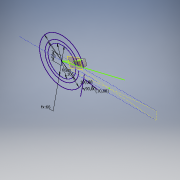
# Autodesk Inventor part: end_stop_plug_v3
Saved by Autodesk Inventor 2016 (Build 200138000, 138)
## iProperties
Created: 2017-11-21
Part Number: end_stop_plug_v3
Material: Generic
Document SubType Name: Modeling
Designer: mbouhier
Density: 1 g/cm^3
Appearance: Default
Author: mbouhier
Autodesk Inventor part; units mm, degrees
ref_plane "YZ Plane" through (0, 0, 0) normal (1, 0, 0) x (0, 1, 0)
ref_plane "XZ Plane" through (0, 0, 0) normal (0, 1, 0) x (-1, 0, 0)
ref_plane "XY Plane" through (0, 0, 0) normal (0, 0, 1) x (1, 0, 0)
sketch "Sketch1" plane through (0, 0, 0) normal (0, 1, 0) x (-1, 0, 0)
  arc A0 (-33, 0) -> (-32.0949, 7.6757) centre (0, 0) ccw
  arc A1 (-40, 0) -> (-38.9029, 9.3039) centre (0, 0) ccw
  arc A2 (-53, 0) -> (-51.5464, 12.3276) centre (0, 0) ccw
  line L0 (-85, 0) -> (100, 0) construction
  line L1 (-226, 10) -> (0, 10) construction
  line L2 (0, 10) -> (0, -10) construction
  line L3 (0, -10) -> (-226, -10) construction
  line L4 (-226, -10) -> (-226, 10) construction
  line L5 (-226, 10) -> (0, -10) construction
  line L6 (0, 10) -> (-226, -10) construction
  line L7 (-52.0481, -10) -> (-44.1646, -51.032)
  line L8 (-38.9029, 9.3039) -> (-32.0949, 7.6757)
  line L9 (-52.0481, -10) -> (-84.6485, -16.2635)
  circle A3 centre (0, 0) radius 33 construction
  line L10 (0, 0) -> (-30.9399, 11.477) construction
  line L11 (-35.5594, 18.3175) -> (-29.3365, 15.1119)
  line L12 (-19.4128, 10) -> (0, 0)
  line L13 (0, 0) -> (-30.5202, 7.2991)
  line L14 (-32.0949, 7.6757) -> (-148.5747, 35.5325)
  line L15 (-35.5594, 18.3175) -> (-47.1162, 24.2707)
  point P0 (-113, 0)
  point P1 (-113, 0)
  point P2 (-45.9257, 26.4544)
  dimension "d13" = 66
  dimension "d0" = 66
  dimension "d1" = 80
  dimension "d2" = 106
  dimension "d3" = 20
  dimension "d5" = 100.876
  dimension "d11" = 90
  dimension "d12" = 10.876
  constraints: 32 end point, 11 point on circle, 9 point on line, 4 coincident, 4 midpoint, 3 centre point, 2 horizontal, 2 parallel, 1 collinear, 1 perpendicular, 1 tangent, 3 other
  measures "d0" diameter of A0
  measures "d1" diameter of A1
  measures "d2" diameter of A2
  measures "d3" distance of L1.end L2.end
  measures "d5" angle of L3 L7
  measures "d11" angle of L9 L7
  measures "d12" angle of L9 L3
extrude "Extrusion1" add sketch "Sketch1" along normal blind 10
sketch "Sketch3" plane through (0, 10, 0) normal (0, 1, 0) x (1, 0, 0)
  line L0 (29.3365, -15.1119) -> (47.1162, -24.2707) projected
  arc A0 (29.3365, -15.1119) -> (32.0949, -7.6757) centre (0, 0) ccw projected
  line L1 (51.5464, -12.3276) -> (32.0949, -7.6757) projected
  arc A1 (47.1162, -24.2707) -> (51.5464, -12.3276) centre (0, 0) ccw projected
  arc A2 (40, 0) -> (38.9029, -9.3039) centre (0, 0) ccw projected
  point P0 (35.5594, -18.3175)
extrude "Extrusion3" cut sketch "Sketch3" against normal blind 2
ref_plane "Work Plane1" through (30.9399, 0, 11.477) normal (0, -1, 0) x (-0.3478, 0, 0.9376)
sketch "Sketch5" plane through (0, 0, 0) normal (0, -1, 0) x (1, 0, 0)
  arc A0 (32.0949, 7.6757) -> (29.3365, 15.1119) centre (0, 0) ccw projected
  arc A1 (29.3365, 15.1119) -> (32.0949, 7.6757) centre (32.0126, 11.8749) ccw
  dimension "d38" = 4.2
  constraints: 2 point on circle, 1 centre point
  measures "d38" radius of A1
extrude "Extrusion5" add sketch "Sketch5" against normal up to surface (8 mm away)
hole "Hole3" at (30.9399, 0, 11.477) direction (0, 1, 0) diameter 3.5 depth 8 tip angle 118 countersink diameter 6 countersink angle 90
equation "\"d13\" = d0"
equation "\"d15\" = 0.5 * d14"
body "Solid1"
